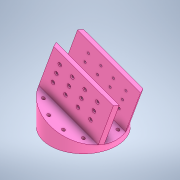
# Autodesk Inventor part: bracketForGarageUpperHalfV02
Saved by Autodesk Inventor 2022.2 (Build 262287000, 287)
## iProperties
Created: 2021-10-20
Part Number: bracketForGarageUpperHalfV02
Material: PC/ABS Plastic
Document SubType Name: Modeling
Designer: robst
Density: 0.357273 g/cm^3
Appearance: Pink
Author: robst
Autodesk Inventor part; units mm, degrees
ref_plane "YZ Plane" through (0, 0, 0) normal (1, 0, 0) x (0, 1, 0)
ref_plane "XZ Plane" through (0, 0, 0) normal (0, 1, 0) x (-1, 0, 0)
ref_plane "XY Plane" through (0, 0, 0) normal (0, 0, 1) x (1, 0, 0)
sketch "Sketch60" plane through (0, 0, 0) normal (0, 1, 0) x (-1, 0, 0)
  circle A0 centre (0, 0) radius 63.5
  dimension "d334" = 127
  constraints: 1 centre point, 1 coincident
  measures "d334" diameter of A0
extrude "Extrusion31" add sketch "Sketch60" against normal blind 10
sketch "Sketch61" plane through (0, 0, 0) normal (0, 1, 0) x (1, 0, 0)
  point P0 (0, 0)
sketch "Sketch62" plane through (0, 0, 0) normal (0, 0, 1) x (1, 0, 0)
  line L0 (63.5, 0) -> (-63.5, 0) projected
  line L1 (-63.5, 0) -> (-63.5, 46.2242)
  line L2 (-63.5, 46.2242) -> (63.5, 0)
  line L3 (-63.5, 0) -> (63.5, 0)
  point P0 (0, 0)
  dimension "d337" = 20
  constraints: 6 end point, 1 perpendicular, 1 vertical
  measures "d337" angle of L2 L0
extrude "Extrusion32" add sketch "Sketch62" along normal up to surface round surface about axis through (0, 0, 0) along (0, -1, 0) radius 63.5 far side no
mirror "Mirror4" about plane through (0, 0, 0) normal (0, 0, 1) of "Extrusion32"
sketch "Sketch63" plane through (0, 23.1121, 0) normal (0.3420201, 0.9396926, 0) x (0.9396926, -0.3420201, 0)
  ellipse E0 centre (0, 0) end of major axis (-67.5753, 0) minor radius 63.5 projected
  line L0 (-60.4826, -28.32) -> (60.4826, -28.32)
  line L1 (-64.022, -20.32) -> (64.022, -20.32)
  line L2 (-64.022, 20.32) -> (64.022, 20.32)
  line L3 (-60.4826, 28.32) -> (60.4826, 28.32)
  ellipse E1 centre (0, 0) end of major axis (0, 63.5) minor radius 67.5753 (-64.022, -20.32) -> (-60.4826, -28.32) ccw
  ellipse E2 centre (0, 0) end of major axis (0, 63.5) minor radius 67.5753 (-60.4826, 28.32) -> (-64.022, 20.32) ccw
  ellipse E3 centre (0, 0) end of major axis (0, 63.5) minor radius 67.5753 (60.4826, -28.32) -> (64.022, -20.32) ccw
  ellipse E4 centre (0, 0) end of major axis (0, 63.5) minor radius 67.5753 (64.022, 20.32) -> (60.4826, 28.32) ccw
  point P0 (7.9048, 0)
  dimension "d340" = 8
  dimension "d341" = 40.64
  constraints: 8 end point, 3 horizontal, 3 parallel, 1 coincident, 25 other
  measures "d340" distance between parallel lines of L0 L1
  measures "d341" distance between parallel lines of L2 L1
sketch "Sketch64" plane through (0, -10, 0) normal (0, -1, 0) x (1, 0, 0)
  circle A0 centre (0, 0) radius 53.975 construction
  line L0 (0, 0) -> (53.975, 0) construction
  line L1 (0, 0) -> (38.1661, -38.1661) construction
  point P0 (52.1358, -13.9698)
  point P1 (52.1358, 13.9698)
  point P2 (38.1661, 38.1661)
  point P3 (13.9698, 52.1358)
  point P4 (-13.9698, 52.1358)
  point P5 (-38.1661, 38.1661)
  point P6 (-52.1358, 13.9698)
  point P7 (-52.1358, -13.9698)
  point P8 (-38.1661, -38.1661)
  point P9 (-13.9698, -52.1358)
  point P10 (13.9698, -52.1358)
  dimension "d342" = 107.95
  dimension "d343" = 45
  dimension "d346" = 360
  constraints: 4 end point, 2 coincident, 2 point on circle, 1 centre point, 1 horizontal, 13 other
  measures "d342" diameter of A0
  measures "d343" angle of L1 L0
hole "Hole13" at (38.1661, -10, -38.1661) at (13.9698, -10, -52.1358) at (-13.9698, -10, -52.1358) at (-38.1661, -10, -38.1661) at (-52.1358, -10, -13.9698) at (-13.9698, -10, 52.1358) at (13.9698, -10, 52.1358) at (38.1661, -10, 38.1661) at (52.1358, -10, 13.9698) at (52.1358, -10, -13.9698) at (-52.1358, -10, 13.9698) at (-38.1661, -10, 38.1661) direction (0, 1, 0) diameter 5.613 end through all clearance for "Flat Head Machine Screw (82)" size "#10" standard "Ansi Unified Screw Threads"
extrude "Extrusion33" add sketch "Sketch63" along normal blind 84.1375 contours L1 E0 L0 | E0 L3 L2
hole "Hole14" at (38.1661, -10, 38.1661) at (-13.9698, -10, 52.1358) at (-38.1661, -10, 38.1661) at (13.9698, -10, 52.1358) at (-52.1358, -10, 13.9698) at (-52.1358, -10, -13.9698) at (-38.1661, -10, -38.1661) at (-13.9698, -10, -52.1358) at (13.9698, -10, -52.1358) at (38.1661, -10, -38.1661) at (52.1358, -10, -13.9698) at (52.1358, -10, 13.9698) direction (0, 1, 0) diameter 6.3246 depth 9.525 counterbore diameter 7.0891 counterbore depth 7.4092
sketch "Sketch65" plane through (-56.8351, 43.7984, 28.32) normal (0, 0, 1) x (0.9396926, -0.3420201, 0)
  line L0 (0, 84.1375) -> (120.9653, 84.1375) projected
  line L1 (0, 0) -> (0, 84.1375) projected
  point P0 (68.3874, -21.7183)
  point P1 (19.05, 65.0875)
  dimension "d364" = 19.05
  dimension "d365" = 19.05
  measures "d364" distance from line of point (19.05, 65.087) L0
  measures "d365" distance from line of point (19.05, 65.087) L1
hole "Hole15" at (-16.6727, 98.4452, 28.32) direction (0, 0, -1) diameter 4.305 depth 8 countersink diameter 7.087 countersink angle 82 clearance for "Flat Head Machine Screw (82)" size "#6" standard "Ansi Unified Screw Threads"
pattern_linear "Rectangular Pattern3" count 4 spacing 25.4 along (0.9396926, -0.3420201, 0) count 3 spacing 19.05 along (-0.3420201, -0.9396926, 0) of "Hole15"
sketch "Sketch67" plane through (56.8351, 2.4258, -28.32) normal (0, 0, -1) x (-0.9396926, 0.3420201, 0)
  line L0 (0, 84.1375) -> (120.9653, 84.1375) projected
  line L1 (0, 0) -> (0, 84.1375) projected
  point P0 (52.5778, -21.7183)
  point P1 (19.05, 65.0875)
  dimension "d379" = 19.05
  dimension "d380" = 19.05
  measures "d379" distance from line of point (19.05, 65.087) L0
  measures "d380" distance from line of L1 point (19.05, 65.087)
hole "Hole16" at (61.1952, 70.1036, -28.32) direction (0, 0, 1) diameter 4.305 depth 8 countersink diameter 7.087 countersink angle 82 clearance for "Flat Head Machine Screw (82)" size "#6" standard "Ansi Unified Screw Threads"
pattern_linear "Rectangular Pattern4" count 4 spacing 25.4 along (-0.9396926, 0.3420201, 0) count 3 spacing 19.05 along (-0.3420201, -0.9396926, 0) of "Hole16"
equation "\"wallThickness\" = 8"
equation "\"twoByFourWidth\" = 40.64"
equation "\"twoByFourDepth\" = 84.1375"
equation "\"azimuth\" = -15deg"
equation "\"elevation\" = 20deg"
equation "\"centerForTwoHoles\" = 0.25 * diagonalLine"
equation "\"depthOfExtrusionForMatingToLowerHalf\" = 12.5"
equation "\"depthForWasherForMatingToCase\" = 14"
equation "\"outsideDiameter\" = 5"
equation "\"diagonalLine\" = 85.134222"
body "Solid4"
body "Solid5"
